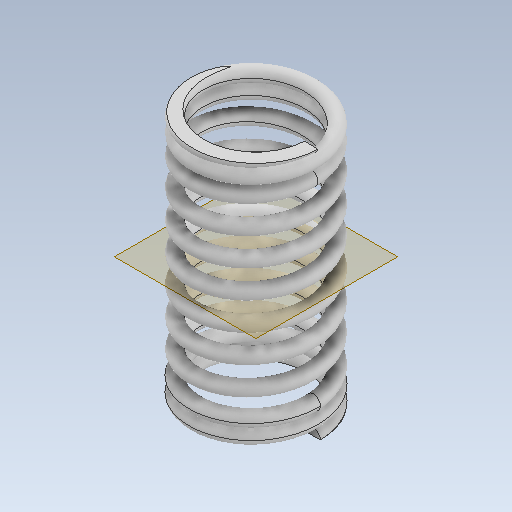
# Autodesk Inventor part: Peça17
Saved by Autodesk Inventor 2021 (Build 250183000, 183)
## iProperties
Category: 41
Created: 2021-07-19
Part Number: Peça17
Material: Genérico
Document SubType Name: Modeling
Designer: Giovanni
Density: 1 g/cm^3
Appearance: Padrão
User Status: 2:1
Author: Giovanni
Keywords: 16
Autodesk Inventor part; units mm, degrees
ref_plane "YZ Plane" through (0, 0, 0) normal (1, 0, 0) x (0, 1, 0)
ref_plane "XY Plane" through (0, 0, 0) normal (0, 0, 1) x (1, 0, 0)
sketch "Esboço1" plane through (0, 0, 0) normal (0, 0, 1) x (1, 0, 0)
  line L0 (0, 0) -> (0, 32.6)
  circle A0 centre (7.4, 0) radius 0.9
  dimension "d0" = 32.6
  dimension "d1" = 1.8
  dimension "d2" = 7.4
  constraints: 2 end point, 1 centre point, 1 horizontal alignment, 1 vertical
  measures "d0" distance of L0.start L0.end
  measures "d1" diameter of A0
  measures "d2" distance of L0.start A0.centre
coil "Espiral1" sketch "Esboço1" operation add axis through (0, 0, 0) along (0, 1, 0) pitch 1.9 turns 2 hand right
sketch "Esboço2" plane through (7.4, 3.8, 0) normal (0, 0, -1) x (-1, 0, 0)
  circle A0 centre (0, 0) radius 0.9 projected
  point P0 (7.4, -3.8)
  point P1 (-0.9, 0)
  constraints: 1 horizontal alignment
coil "Espiral2" sketch "Esboço2" operation add axis through (0, -10, 0) along (0, 1, 0) pitch 3.6 turns 6.994 hand right
sketch "Esboço3" plane through (7.3947, 28.9784, 0.2789) normal (0.0377, 0, -0.9993) x (-0.9993, 0, -0.0377)
  circle A0 centre (0, 0) radius 0.9 projected
  point P0 (7.4, -28.9784)
  point P1 (0.9, 0)
  constraints: 1 horizontal alignment
coil "Espiral3" sketch "Esboço3" operation add axis through (0, -10, 0) along (0, 1, 0) pitch 1.9 turns 2 hand right
sketch "Esboço4" plane through (0, 0, 0) normal (0, 1, 0) x (-1, 0, 0)
  line L0 (13, -12) -> (-12, -12)
  line L1 (-12, -12) -> (-12, 13)
  line L2 (-12, 13) -> (13, 13)
  line L3 (13, 13) -> (13, -12)
  point P0 (0, 0)
  dimension "d27" = 25
  dimension "d28" = 25
  dimension "d29" = 13
  dimension "d30" = 13
  constraints: 8 end point, 2 parallel, 1 horizontal, 1 perpendicular
  measures "d27" distance of L1.end L2.end
  measures "d28" distance of L0.end L1.end
  measures "d29" vertical distance of L1.end point (0, 0)
  measures "d30" distance from line of point (0, 0) L3
extrude "Extrusão1" cut sketch "Esboço4" against normal blind 5
ref_plane "Plano de trabalho1" through (0, 16.3, 0) normal (0, 1, 0) x (-1, 0, 0)
mirror "Espelhamento1" about plane through (0, 16.3, 0) normal (0, 1, 0) of "Extrusão1"
